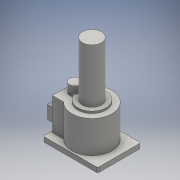
# Autodesk Inventor part: Base
Saved by Autodesk Inventor 2016 (Build 200138000, 138)
## iProperties
Created: 2015-12-17
Part Number: Base
Material: Generic
Document SubType Name: Modeling
Designer: ajshort
Density: 1 g/cm^3
Appearance: Default
Author: ajshort
Autodesk Inventor part; units mm, degrees
ref_plane "YZ Plane" through (0, 0, 0) normal (1, 0, 0) x (0, 1, 0)
ref_plane "XZ Plane" through (0, 0, 0) normal (0, 1, 0) x (-1, 0, 0)
ref_plane "XY Plane" through (0, 0, 0) normal (0, 0, 1) x (1, 0, 0)
sketch "Sketch1" plane through (0, 0, 0) normal (0, 0, 1) x (1, 0, 0)
  line L0 (-241.5, 190.5) -> (241.5, 190.5)
  line L1 (241.5, 190.5) -> (241.5, -190.5)
  line L2 (241.5, -190.5) -> (-241.5, -190.5)
  line L3 (-241.5, -190.5) -> (-241.5, 190.5)
  point P0 (0, 0)
  point P1 (241.5, 0)
  point P2 (0, 190.5)
  dimension "d0" = 483
  dimension "d1" = 381
  constraints: 8 end point, 2 midpoint, 2 parallel, 1 horizontal, 1 horizontal alignment, 1 perpendicular, 1 vertical alignment
  measures "d0" distance of L0.start L0.end
  measures "d1" distance of L2.end L0.start
extrude "Extrusion1" add sketch "Sketch1" along normal blind 43.2
fillet "Fillet1" radius 12.7 4 edges at (241.5, 190.5, 21.6) (-241.5, 190.5, 21.6) (241.5, -190.5, 21.6) (-241.5, -190.5, 21.6)
sketch "Sketch2" plane through (0, 0, 43.2) normal (0, 0, 1) x (1, 0, 0)
  circle A0 centre (0, 0) radius 177.5 construction
  line L0 (-225, 124) -> (-225, -124)
  line L1 (-225, 124) -> (-127.0049, 124)
  line L2 (-241.5, -177.8) -> (-241.5, 177.8) projected
  line L3 (-225, -124) -> (-127.0049, -124)
  arc A1 (-127.0049, -124) -> (-127.0049, 124) centre (0, 0) ccw
  point P0 (-225, 0)
  dimension "d5" = 355
  dimension "d6" = 248
  dimension "d7" = 225
  constraints: 6 end point, 4 point on circle, 2 centre point, 2 coincident, 1 horizontal, 1 horizontal alignment, 1 midpoint, 1 perpendicular, 1 vertical
  measures "d5" diameter of A0
  measures "d6" distance of L0.start L0.end
  measures "d7" distance from line of point (0, 0) L0
extrude "Extrusion2" add sketch "Sketch2" along normal blind 286.8
sketch "Sketch3" plane through (-225, -124, 43.2) normal (-1, 0, 0) x (0, 0, 1)
  line L0 (191.2, 243) -> (74.2, 243)
  line L1 (74.2, 243) -> (74.2, 5)
  line L2 (74.2, 5) -> (191.2, 5)
  line L3 (191.2, 5) -> (191.2, 243)
  line L4 (0, 301.8) -> (0, -53.8) projected
  point P0 (-43.2, 124)
  point P1 (191.2, 124)
  point P2 (0, 124)
  dimension "d10" = 238
  dimension "d11" = 117
  dimension "d12" = 74.2
  constraints: 8 end point, 2 midpoint, 2 parallel, 1 horizontal, 1 horizontal alignment, 1 perpendicular
  measures "d10" distance of L2.end L0.start
  measures "d11" distance of L0.start L0.end
  measures "d12" distance between parallel lines of L4 L1
extrude "Extrusion3" add sketch "Sketch3" along normal blind 51
sketch "Sketch4" plane through (0, 0, 330) normal (0, 0, 1) x (1, 0, 0)
  circle A0 centre (0, 0) radius 125 construction
  circle A1 centre (-150, 0) radius 48.5 construction
  line L0 (-150, 48.5) -> (-115.2074, 48.5)
  line L1 (-150, -48.5) -> (-115.2074, -48.5)
  arc A2 (-150, 48.5) -> (-150, -48.5) centre (-150, 0) ccw
  arc A3 (-115.2074, -48.5) -> (-115.2074, 48.5) centre (0, 0) ccw
  dimension "d15" = 250
  dimension "d16" = 97
  dimension "d17" = 150
  constraints: 8 point on circle, 4 centre point, 4 end point, 3 coincident, 2 horizontal, 1 horizontal alignment, 1 parallel, 1 tangent
  measures "d15" diameter of A0
  measures "d16" diameter of A1
  measures "d17" distance of point (0, 0) A1.centre
extrude "Extrusion4" add sketch "Sketch4" along normal blind 19
sketch "Sketch5" plane through (0, 0, 349) normal (0, 0, 1) x (1, 0, 0)
  arc A0 (-150, 48.5) -> (-150, -48.5) centre (-150, 0) ccw projected
  circle A1 centre (-150, 0) radius 48.5
  point P0 (0, 0)
  constraints: 1 coincident, 1 vertical alignment, 2 other
extrude "Extrusion5" add sketch "Sketch5" along normal blind 64
sketch "Sketch6" plane through (0, 0, 349) normal (0, 0, 1) x (1, 0, 0)
  circle A0 centre (0, 0) radius 84
  dimension "d22" = 168
  constraints: 1 centre point, 1 coincident
  measures "d22" diameter of A0
extrude "Extrusion6" add sketch "Sketch6" along normal blind 479
body "Solid1"
